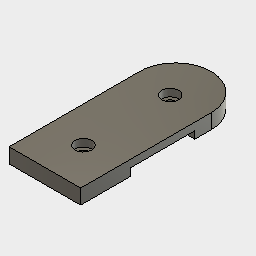
Butterfly Switch Clip (Autodesk Fusion 360 design; units mm, degrees)
Autodesk Fusion 360 part; units mm, degrees
sketch "Base Outline" plane through (0, 0, 0) normal (0, 1, 0) x (1, 0, 0)
  line L0 (0, 0) -> (19.3, 0)
  line L1 (19.3, 0) -> (19.3, 35.2)
  line L2 (19.3, 35.2) -> (0, 35.2)
  line L3 (0, 35.2) -> (0, 0)
  arc A0 (19.3, 35.2) -> (0, 35.2) centre (9.65, 35.2) ccw
  dimension "d1" = 19.3
  dimension "d2" = 35.2
  constraint horizontal L0
  constraint vertical L1
  constraint horizontal L2
  constraint vertical L3
  constraint midpoint L2
extrude "Extrude1" add sketch "Base Outline" along normal blind 4
sketch "Mounting Holes" plane through (0, 4, 0) normal (0, 1, 0) x (-1, 0, 0)
  line L0 (0, 0) -> (-19.3, 0)
  arc A0 (-19.3, -35.2) -> (0, -35.2) centre (-9.65, -35.2) ccw
  line L1 (-9.65, 0) -> (-9.65, -44.85) construction
  circle A1 centre (-9.65, -10.375) radius 1.25
  circle A2 centre (-9.65, -33.825) radius 1.25
  dimension "d50" = 10.375
  dimension "d51" = 23.45
  dimension "d52" = 2.5
  constraint midpoint L0
  constraint midpoint A0
  constraint coincident L1
  constraint equal A1 A2
  measures "d50" distance of L0
  measures "d52" diameter of A2
extrude "Extrude11" cut sketch "Mounting Holes" against normal blind 5
sketch "Mounting Hole Countersinks" plane through (0, 4, 0) normal (0, 1, 0) x (-1, 0, 0)
  circle A0 centre (-9.65, -10.375) radius 1.25
  circle A1 centre (-9.65, -33.825) radius 1.25
  arc A2 (-19.3, -35.2) -> (0, -35.2) centre (-9.65, -35.2) ccw
  line L0 (0, -35.2) -> (0, 0)
  line L1 (0, 0) -> (-19.3, 0)
  line L2 (-19.3, 0) -> (-19.3, -35.2)
  circle A3 centre (-9.65, -33.825) radius 2.25
  circle A4 centre (-9.65, -10.375) radius 2.25
  dimension "d55" = 4.5
  constraint concentric A1 A3
  constraint concentric A0 A4
  constraint equal A3 A4
  measures "d55" diameter of A3
extrude "Extrude12" cut sketch "Mounting Hole Countersinks" against normal blind 2 contours A3 | A4
sketch "Strap Cutout" plane through (0, 0, 0) normal (0, 1, 0) x (1, 0, 0)
  line L0 (0, 30.825) -> (19.3, 30.825)
  line L1 (19.3, 30.825) -> (19.3, 13.375)
  line L2 (19.3, 13.375) -> (0, 13.375)
  line L3 (0, 13.375) -> (0, 30.825)
  line L4 (0, 35.2) -> (0, 0)
  line L5 (0, 35.2) -> (0, 0)
  line L6 (19.3, 0) -> (19.3, 35.2)
  line L7 (19.3, 0) -> (19.3, 35.2)
  line L8 (0, 0) -> (19.3, 0)
  arc A0 (19.3, 35.2) -> (0, 35.2) centre (9.65, 35.2) ccw
  dimension "d62" = 17.45
  dimension "d63" = 13.375
  dimension "d64" = 14.025
  constraint horizontal L0
  constraint vertical L1
  constraint horizontal L2
  constraint vertical L3
  constraint coincident L6
  constraint coincident L4
  constraint midpoint A0
  measures "d63" distance of L2 L8
  measures "d64" distance of L0
extrude "Extrude13" cut sketch "Strap Cutout" along normal blind 2 contours L0 L1 L2 L3 L4 L5 L6 L7
